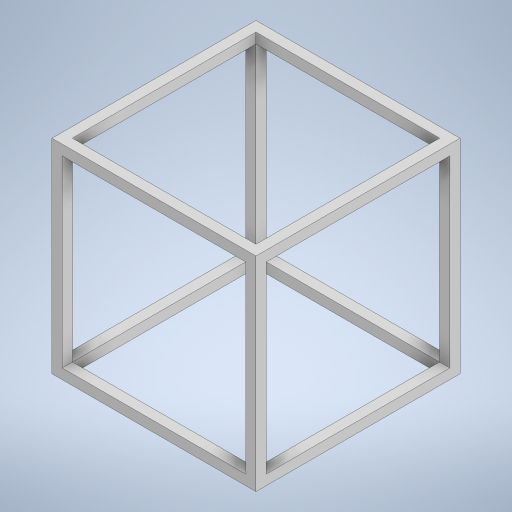
# Autodesk Inventor part: wymiar
Saved by Autodesk Inventor 2023.5 (Build 275446000, 446)
## iProperties
Created: 2025-03-16
Part Number: wymiar
Material: Ogólny
Document SubType Name: Modeling
Designer: kamil
Density: 1 g/cm^3
Appearance: Domyślna
Author: kamil
Autodesk Inventor part; units mm, degrees
ref_plane "YZ Plane" through (0, 0, 0) normal (1, 0, 0) x (0, 1, 0)
ref_plane "XZ Plane" through (0, 0, 0) normal (0, 1, 0) x (-1, 0, 0)
ref_plane "XY Plane" through (0, 0, 0) normal (0, 0, 1) x (1, 0, 0)
sketch "Szkic1" plane through (0, 0, 0) normal (1, 0, 0) x (0, 1, 0)
  line L0 (0, 0) -> (100, 0)
  line L1 (100, 0) -> (100, -100)
  line L2 (100, -100) -> (0, -100)
  line L3 (0, -100) -> (0, 0)
  line L4 (95, -95) -> (95, -5)
  line L5 (95, -5) -> (5, -5)
  line L6 (5, -5) -> (5, -95)
  line L7 (5, -95) -> (95, -95)
  dimension "d0" = 100
  dimension "d1" = 100
  dimension "d2" = 5
  constraints: 16 end point, 4 parallel, 2 perpendicular, 1 horizontal, 3 other
  measures "d0" distance of L1.end L2.end
  measures "d1" distance of L0.end L1.end
  measures "d2" distance between parallel lines of L1 L4
extrude "Wyciągnięcie proste1" add sketch "Szkic1" along normal blind 5
sketch "Szkic2" plane through (5, 0, 0) normal (1, 0, 0) x (0, 0, -1)
  line L0 (100, 0) -> (100, 100) projected
  line L1 (100, 100) -> (0, 100) projected
  line L2 (0, 100) -> (0, 0) projected
  line L3 (0, 0) -> (100, 0) projected
  line L4 (95, 95) -> (95, 5) projected
  line L5 (95, 5) -> (5, 5) projected
  line L6 (5, 5) -> (5, 95) projected
  line L7 (5, 95) -> (95, 95) projected
  line L8 (0, 100) -> (5, 100)
  line L9 (5, 100) -> (5, 95)
  line L10 (5, 95) -> (0, 95)
  line L11 (0, 95) -> (0, 100)
  line L12 (5, 95) -> (95, 95) projected
  line L13 (100, 100) -> (95, 100)
  line L14 (95, 100) -> (95, 95)
  line L15 (95, 95) -> (100, 95)
  line L16 (100, 95) -> (100, 100)
  line L17 (95, 95) -> (95, 5) projected
  line L18 (95, 5) -> (100, 5)
  line L19 (100, 5) -> (100, 0)
  line L20 (100, 0) -> (95, 0)
  line L21 (95, 0) -> (95, 5)
  line L22 (5, 5) -> (5, 95) projected
  line L23 (0, 100) -> (0, 0) projected
  line L24 (5, 5) -> (0, 5)
  line L25 (0, 5) -> (0, 0)
  line L26 (0, 0) -> (5, 0)
  line L27 (5, 0) -> (5, 5)
  constraints: 32 end point, 8 parallel, 4 horizontal, 4 perpendicular
extrude "Wyciągnięcie proste2" add sketch "Szkic2" along normal blind 90 contours L3 L21 L18 L0 | L15 L14 L1 L0 | L3 L2 L24 L27 | L10 L2 L1 L9
sketch "Szkic3" plane through (95, 0, 0) normal (1, 0, 0) x (0, 0, -1)
  line L0 (100, 0) -> (100, 100) projected
  line L1 (0, 0) -> (100, 0) projected
  line L2 (0, 100) -> (0, 0) projected
  line L3 (100, 100) -> (0, 100) projected
  line L4 (95, 95) -> (95, 5) projected
  line L5 (5, 95) -> (95, 95) projected
  line L6 (5, 5) -> (5, 95) projected
  line L7 (95, 5) -> (5, 5) projected
extrude "Wyciągnięcie proste3" add sketch "Szkic3" along normal blind 5
